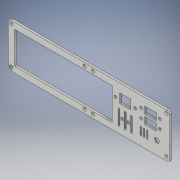
# Autodesk Inventor part: CyberDeckIOPanel2
Saved by Autodesk Inventor 2019.4 (Build 234330000, 330)
## iProperties
Created: 2020-07-26
Part Number: CyberDeckIOPanel2
Material: Generic
Document SubType Name: Modeling
Designer: Briti
Density: 1 g/cm^3
Appearance: Default
Author: Briti
Autodesk Inventor part; units mm, degrees
ref_plane "YZ Plane" through (0, 0, 0) normal (1, 0, 0) x (0, 1, 0)
ref_plane "XZ Plane" through (0, 0, 0) normal (0, 1, 0) x (-1, 0, 0)
ref_plane "XY Plane" through (0, 0, 0) normal (0, 0, 1) x (1, 0, 0)
sketch "Sketch1" plane through (0, 0, 0) normal (0, 0, 1) x (1, 0, 0)
  line L0 (-116.5, -32) -> (116.5, -32)
  line L1 (116.5, -32) -> (116.5, 32)
  line L2 (116.5, 32) -> (-116.5, 32)
  line L3 (-116.5, 32) -> (-116.5, -32)
  line L4 (-116.5, -32) -> (116.5, 32) construction
  line L5 (116.5, -32) -> (-116.5, 32) construction
  point P0 (0, 0)
  dimension "d0" = 233
  dimension "d1" = 64
  constraints: 12 end point, 2 midpoint, 2 parallel, 1 horizontal, 1 perpendicular
  measures "d0" distance of L2.end L1.end
  measures "d1" distance of L0.end L1.end
extrude "Extrusion1" add sketch "Sketch1" along normal blind 3
sketch "Sketch2" plane through (0, 0, 3) normal (0, 0, 1) x (1, 0, 0)
  arc A0 (-112, 32) -> (-116.5, 27.5) centre (-112, 27.5) ccw
  line L0 (116.5, 32) -> (-116.5, 32) projected
  line L1 (-116.5, 32) -> (-116.5, -32) projected
  arc A1 (116.5, 27.5) -> (112, 32) centre (112, 27.5) ccw
  line L2 (116.5, -32) -> (116.5, 32) projected
  line L3 (-112, 27.5) -> (-112, -26.5) construction
  line L4 (-116.5, -32) -> (116.5, -32) construction
  line L5 (-112, -26.5) -> (-107.482, -26.5) construction
  line L6 (-107.482, -26.5) -> (-107.482, -22) construction
  line L7 (-107.5, -22) -> (107.5, -22) construction
  line L8 (107.5, -22) -> (107.5, 23) construction
  line L9 (107.5, 23) -> (-107.5, 23) construction
  line L10 (-107.5, 23) -> (-107.5, -22) construction
  line L11 (-107.5, -22) -> (107.5, 23) construction
  line L12 (107.5, -22) -> (-107.5, 23) construction
  point P0 (0, 0)
  point P1 (0, 0.5)
  dimension "d4" = 9
  dimension "d5" = 9
  dimension "d6" = 54
  dimension "d7" = 4.518
  dimension "d8" = 4.5
  dimension "d9" = 215
  dimension "d10" = 45
  dimension "d11" = 9
  dimension "d12" = 9
  dimension "d13" = 9
  constraints: 18 end point, 4 point on circle, 4 point on line, 4 tangent, 2 centre point, 2 horizontal, 2 midpoint, 2 parallel, 2 perpendicular, 1 vertical
  measures "d4" diameter of A0
  measures "d5" diameter of A1
  measures "d6" distance of L3.start L3.end
  measures "d7" distance of L3.end L5.end
  measures "d8" distance of L5.end L6.end
  measures "d9" distance of L9.end L8.end
  measures "d10" distance of L8.end L7.end
  measures "d11" distance between parallel lines of L2 L8
  measures "d12" distance between parallel lines of L10 L1
  measures "d13" distance between parallel lines of L9 L0
extrude "Extrusion2" cut sketch "Sketch2" against normal blind 5
sketch "Sketch6" plane through (0, 0, 3) normal (0, 0, 1) x (1, 0, 0)
  line L0 (107.5, -22) -> (-107.5, -22) construction
  line L1 (-107.5, -22) -> (-116.5, -22) construction
  line L2 (-116.5, 27.5) -> (-116.5, -32) construction
  line L3 (-107.5, -22) -> (-107.5, -32) construction
  line L4 (-116.5, -32) -> (116.5, -32) construction
  arc A0 (-116.5, -27) -> (-111.5, -32) centre (-111.5, -27) ccw
  line L5 (-111.5, -32) -> (-116.5, -32)
  line L6 (-116.5, -32) -> (-116.5, -27)
  point P0 (0, 0)
  dimension "d32" = 10
  constraints: 8 end point, 4 point on line, 2 perpendicular, 2 point on circle, 2 tangent, 1 centre point, 1 collinear, 1 horizontal
  measures "d32" diameter of A0
extrude "Extrusion6" cut sketch "Sketch6" against normal blind 5
sketch "Sketch7" plane through (0, 0, 3) normal (0, 0, 1) x (1, 0, 0)
  arc A0 (-112, 32) -> (-116.5, 27.5) centre (-112, 27.5) ccw projected
  circle A1 centre (-112, 27.5) radius 2.4
  arc A2 (116.5, 27.5) -> (112, 32) centre (112, 27.5) ccw projected
  circle A3 centre (112, 27.5) radius 2.4
  point P0 (0, 0)
  dimension "d35" = 4.8
  dimension "d36" = 4.8
  constraints: 2 centre point, 2 coincident
  measures "d35" diameter of A1
  measures "d36" diameter of A3
extrude "Extrusion7" cut sketch "Sketch7" against normal blind 5
sketch "Sketch8" plane through (0, 0, 3) normal (0, 0, 1) x (1, 0, 0)
  arc A0 (-116.5, -27) -> (-111.5, -32) centre (-111.5, -27) ccw construction
  line L0 (-116.5, -27) -> (-116.5, -23.25) construction
  line L1 (-116.5, 27.5) -> (-116.5, -27) construction
  line L2 (-111.5, -32) -> (-107.75, -32) construction
  line L3 (-111.5, -32) -> (116.5, -32) construction
  arc A1 (-116.5, -23.25) -> (-107.75, -32) centre (-106.5699, -22.0699) ccw
  line L4 (-116.5, -23.25) -> (-116.5, -27)
  line L5 (-107.75, -32) -> (-111.5, -32)
  arc A2 (-116.5, -27) -> (-111.5, -32) centre (-111.5, -27) ccw
  point P0 (0, 0)
  dimension "d39" = 3.75
  dimension "d40" = 3.75
  dimension "d41" = 10
  constraints: 8 end point, 4 point on circle, 2 centre point, 2 collinear, 2 point on line, 1 concentric
  measures "d39" distance of L0.start L0.end
  measures "d40" distance of L2.start L2.end
  measures "d41" radius of A1
extrude "Extrusion8" cut sketch "Sketch8" against normal blind 5
sketch "Sketch9" plane through (0, 0, 3) normal (0, 0, 1) x (1, 0, 0)
  line L0 (-107.5, -22) -> (107.5, -22) construction
  line L1 (107.5, -22) -> (107.5, -32) construction
  line L2 (-107.75, -32) -> (116.5, -32) construction
  line L3 (107.5, -22) -> (120.5, -22) construction
  line L4 (107.5, -32) -> (111.5, -32) construction
  line L5 (120.5, -22) -> (120.5, -23) construction
  arc A0 (111.5, -32) -> (120.5, -23) centre (110.5456, -22.0456) ccw construction
  line L6 (116.5, -32) -> (116.5, 27.5) projected
  arc A1 (111.5, -32) -> (116.5, -30.0797) centre (110.5456, -22.0456) ccw
  line L7 (116.5, -30.0797) -> (116.5, -32)
  line L8 (111.5, -32) -> (116.5, -32)
  point P0 (0, 0)
  dimension "d44" = 13
  dimension "d45" = 4
  dimension "d46" = 1
  dimension "d47" = 10
  constraints: 12 end point, 5 point on circle, 3 point on line, 2 centre point, 2 collinear, 2 vertical, 1 concentric, 1 perpendicular
  measures "d44" distance of L0.end L3.end
  measures "d45" distance of L1.end L4.end
  measures "d46" distance of L3.end L5.end
  measures "d47" radius of A0
extrude "Extrusion9" cut sketch "Sketch9" against normal blind 5
sketch "Sketch10" plane through (0, 0, 3) normal (0, 0, 1) x (1, 0, 0)
  circle A0 centre (5.75, 27.5) radius 2.4
  line L0 (112, 32) -> (-112, 32) projected
  line L1 (-107.5, 23) -> (107.5, 23) projected
  circle A1 centre (112, 27.5) radius 2.4 projected
  circle A2 centre (-6.25, 27.5) radius 2.4
  circle A3 centre (5.75, -26.5) radius 2.4
  circle A4 centre (-6.25, -26.5) radius 2.4
  point P0 (0, 0)
  dimension "d50" = 4.8
  dimension "d51" = 4.5
  dimension "d52" = 4.5
  dimension "d53" = 106.25
  dimension "d54" = 4.8
  dimension "d55" = 12
  dimension "d56" = 4.8
  dimension "d57" = 54
  dimension "d58" = 4.8
  dimension "d59" = 12
  constraints: 4 centre point, 2 horizontal alignment, 1 vertical alignment
  measures "d50" diameter of A0
  measures "d51" distance from line of L0 A0.centre
  measures "d52" distance from line of L1 A0.centre
  measures "d53" distance of A1.centre A0.centre
  measures "d54" diameter of A2
  measures "d55" distance of A0.centre A2.centre
  measures "d56" diameter of A3
  measures "d57" distance of A3.centre A0.centre
  measures "d58" diameter of A4
  measures "d59" distance of A3.centre A4.centre
extrude "Extrusion10" cut sketch "Sketch10" against normal blind 5 contours A0 | A2 | A3 | A4
sketch "Sketch11" plane through (0, 0, 3) normal (0, 0, 1) x (1, 0, 0)
  circle A0 centre (112, -26.4995) radius 2.4
  circle A1 centre (112, 27.5) radius 2.4 construction
  circle A2 centre (112, 27.5) radius 2.4 construction
  circle A3 centre (112, -26.4995) radius 4.5 construction
  line L0 (-107.5, -22) -> (107.5, -22) construction
  line L1 (107.5, -22) -> (112.0687, -22) construction
  line L2 (107.5, -22) -> (107.5, 23) construction
  line L3 (107.5, -22) -> (107.5, -26.4995) construction
  point P0 (0, 0)
  dimension "d62" = 4.8
  dimension "d63" = 9
  constraints: 4 end point, 3 centre point, 2 coincident, 2 point on circle, 1 collinear, 1 tangent, 1 vertical alignment
  measures "d62" diameter of A0
  measures "d63" diameter of A3
extrude "Extrusion11" cut sketch "Sketch11" against normal blind 5
sketch "Sketch12" plane through (0, 0, 3) normal (0, 0, 1) x (1, 0, 0)
  line L0 (-107.5, -22) -> (107.5, -22) construction
  line L1 (-107.5, -22) -> (-116.5, -22) construction
  line L2 (-116.5, 27.5) -> (-116.5, -23.25) construction
  arc A0 (-116.5, -23.25) -> (-107.75, -32) centre (-106.5699, -22.0699) ccw construction
  line L3 (-107.5, -22) -> (-107.75, -32) construction
  circle A1 centre (-112.1139, -26.5) radius 4.5 construction
  circle A2 centre (-112.1139, -26.5) radius 2.4
  point P0 (0, 0)
  dimension "d66" = 9
  dimension "d67" = 4.8
  constraints: 4 end point, 2 centre point, 2 tangent, 1 coincident, 1 horizontal, 1 point on line
  measures "d66" diameter of A1
  measures "d67" diameter of A2
extrude "Extrusion12" cut sketch "Sketch12" against normal blind 5
sketch "Sketch22" plane through (0, 0, 0) normal (0, 0, -1) x (-1, 0, 0)
  line L0 (107.75, -32) -> (-111.5, -32) construction
  line L1 (-116.5, 32) -> (-107.5, 32) construction
  line L2 (-107.5, 32) -> (-107.5, -32) construction
  line L3 (-107.5, -32) -> (-116.5, -32) construction
  line L4 (-116.5, -32) -> (-116.5, 32) construction
  line L5 (116.5, 27.5) -> (116.5, -23.25) construction
  line L6 (-116.5, -32) -> (116.5, -32) construction
  line L7 (116.5, -32) -> (116.5, -23) construction
  line L8 (116.5, -23) -> (-116.5, -23) construction
  line L9 (-116.5, -23) -> (-116.5, -32) construction
  line L10 (-112, 32) -> (112, 32) construction
  line L11 (116.5, -32) -> (107.5, -32) construction
  line L12 (107.5, -32) -> (107.5, 32) construction
  line L13 (107.5, 32) -> (116.5, 32) construction
  line L14 (116.5, 32) -> (116.5, -32) construction
  line L15 (-116.5, -30.0797) -> (-116.5, 27.5) construction
  line L16 (116.5, 32) -> (-116.5, 32) construction
  line L17 (-116.5, 32) -> (-116.5, 23) construction
  line L18 (-116.5, 23) -> (116.5, 23) construction
  line L19 (116.5, 23) -> (116.5, 32) construction
  line L20 (-107.5, 23) -> (-107.5, 16) construction
  line L21 (-107.5, 16) -> (-102.5, 16) construction
  circle A0 centre (-102.5, 16) radius 5 construction
  line L22 (-97.5, 16) -> (-80.5, 16) construction
  line L23 (-80.5, 16) -> (-75.5, 16) construction
  circle A1 centre (-75.5, 16) radius 5 construction
  line L24 (-80.5, 10) -> (-97.5, 10) construction
  line L25 (-97.5, 10) -> (-97.5, 22) construction
  line L26 (-97.5, 22) -> (-80.5, 22) construction
  line L27 (-80.5, 22) -> (-80.5, 10) construction
  line L28 (-80.5, 10) -> (-97.5, 22) construction
  line L29 (-97.5, 10) -> (-80.5, 22) construction
  line L30 (-97.5, 22) -> (-99.5, 22) construction
  line L31 (-99.5, 22) -> (-99.5, 10) construction
  line L32 (-99.5, 10) -> (-97.5, 9) construction
  line L33 (-80.5, 22) -> (-78.5, 22) construction
  line L34 (-78.5, 22) -> (-78.5, 10) construction
  line L35 (-78.5, 10) -> (-80.5, 10) construction
  line L36 (-97.5, 11) -> (-80.5, 11)
  line L37 (-80.5, 11) -> (-80.5, 21)
  line L38 (-80.5, 21) -> (-97.5, 21)
  line L39 (-97.5, 21) -> (-97.5, 11)
  line L40 (-97.5, 11) -> (-80.5, 21) construction
  line L41 (-80.5, 11) -> (-97.5, 21) construction
  circle A2 centre (-102.5, 16) radius 2
  circle A3 centre (-75.5, 16) radius 2
  line L42 (-97.5, 9) -> (-80.5, 9) construction
  line L43 (-80.5, 9) -> (-80.5, -3) construction
  line L44 (-80.5, -3) -> (-97.5, -3) construction
  line L45 (-97.5, -3) -> (-97.5, 9) construction
  line L46 (-97.5, 3) -> (-102.5, 3) construction
  line L47 (-80.5, 3) -> (-75.5, 3) construction
  circle A4 centre (-102.5, 3) radius 5 construction
  circle A5 centre (-75.5, 3) radius 5 construction
  line L48 (-97.5, 9) -> (-99.5, 10) construction
  line L49 (-99.5, 10) -> (-99.5, -3) construction
  line L50 (-99.5, -3) -> (-97.5, -3) construction
  line L51 (-80.5, -3) -> (-78.5, -3) construction
  line L52 (-78.5, -3) -> (-78.5, 10) construction
  line L53 (-78.5, 10) -> (-80.5, 10) construction
  line L54 (-89, 9) -> (-89, -3) construction
  line L55 (-97.5, 3) -> (-80.5, 3) construction
  line L56 (-97.5, -2) -> (-80.5, -2)
  line L57 (-80.5, -2) -> (-80.5, 8)
  line L58 (-80.5, 8) -> (-97.5, 8)
  line L59 (-97.5, 8) -> (-97.5, -2)
  line L60 (-97.5, -2) -> (-80.5, 8) construction
  line L61 (-80.5, -2) -> (-97.5, 8) construction
  circle A6 centre (-102.5, 3) radius 2
  circle A7 centre (-75.5, 3) radius 2
  line L62 (-89, -3) -> (-89, -23) construction
  line L63 (-89, -13) -> (-107.5, -13) construction
  line L64 (-70.5, 16) -> (-70.5, 23) construction
  line L65 (-70.5, 16) -> (-70.5, -23) construction
  line L66 (-89, -13) -> (-70.5, -13) construction
  circle A8 centre (-98.25, -13) radius 3.5
  line L67 (-79.75, -18) -> (-79.75, -8) construction
  line L68 (-78.75, -18) -> (-78.75, -8)
  line L69 (-80.75, -8) -> (-80.75, -18)
  arc A9 (-80.75, -18) -> (-78.75, -18) centre (-79.75, -18) ccw
  arc A10 (-78.75, -8) -> (-80.75, -8) centre (-79.75, -8) ccw
  line L70 (-89, -13) -> (-79.75, -13) construction
  line L71 (-79.75, -13) -> (-70.5, -13) construction
  line L72 (-84.375, -18) -> (-84.375, -8) construction
  line L73 (-83.375, -18) -> (-83.375, -8)
  line L74 (-85.375, -8) -> (-85.375, -18)
  arc A11 (-85.375, -18) -> (-83.375, -18) centre (-84.375, -18) ccw
  arc A12 (-83.375, -8) -> (-85.375, -8) centre (-84.375, -8) ccw
  line L75 (-75.125, -18) -> (-75.125, -8) construction
  line L76 (-74.125, -18) -> (-74.125, -8)
  line L77 (-76.125, -8) -> (-76.125, -18)
  arc A13 (-76.125, -18) -> (-74.125, -18) centre (-75.125, -18) ccw
  arc A14 (-74.125, -8) -> (-76.125, -8) centre (-75.125, -8) ccw
  point P0 (0, 0)
  point P1 (-89, 16)
  point P2 (-89, 3)
  point P3 (-84.375, -13)
  point P4 (-75.125, -13)
  dimension "d172" = 9
  dimension "d173" = 9
  dimension "d174" = 9
  dimension "d175" = 9
  dimension "d176" = 7
  dimension "d177" = 5
  dimension "d178" = 17
  dimension "d179" = 5
  dimension "d180" = 12
  dimension "d181" = 2
  dimension "d182" = 2
  dimension "d183" = 17
  dimension "d184" = 10
  dimension "d185" = 4
  dimension "d186" = 4
  dimension "d187" = 12
  dimension "d188" = 5
  dimension "d189" = 5
  dimension "d190" = 2
  dimension "d191" = 17
  dimension "d192" = 10
  dimension "d193" = 4
  dimension "d194" = 4
  dimension "d195" = 7
  dimension "d196" = 5
  dimension "d197" = 2
  dimension "d198" = 5
  dimension "d199" = 2
  dimension "d200" = 5
  dimension "d201" = 2
  dimension "d204" = 37
  constraints: 154 end point, 21 parallel, 20 midpoint, 20 perpendicular, 18 point on line, 16 point on circle, 13 centre point, 13 horizontal, 13 tangent, 8 coincident, 3 collinear, 2 horizontal alignment, 4 other
  measures "d172" distance of L2.end L3.end
  measures "d173" distance of L7.end L6.end
  measures "d174" distance of L12.end L13.end
  measures "d175" distance of L17.end L16.end
  measures "d176" distance of L20.start L20.end
  measures "d177" distance of L20.end L21.end
  measures "d178" distance of L22.start L22.end
  measures "d179" distance of L22.end L23.end
  measures "d180" distance of L24.end L25.end
  measures "d181" distance of L25.end L30.end
  measures "d182" distance of L26.end L33.end
  measures "d183" distance of L38.end L37.end
  measures "d184" distance of L37.end L36.end
  measures "d185" diameter of A2
  measures "d186" diameter of A3
  measures "d187" distance of L42.end L43.end
  measures "d188" distance of L46.start L46.end
  measures "d189" distance of L47.start L47.end
  measures "d190" distance of L43.end L51.end
  measures "d191" distance of L58.end L57.end
  measures "d192" distance of L57.end L56.end
  measures "d193" diameter of A6
  measures "d194" diameter of A7
  measures "d195" diameter of A8
  measures "d196" distance of L70.end L67.end
  measures "d197" diameter of A10
  measures "d198" distance of point (-84.375, -13) L72.end
  measures "d199" diameter of A12
  measures "d200" distance of point (-75.125, -13) L75.end
  measures "d201" diameter of A14
  measures "d204" distance of L20.start L64.end
extrude "Extrusion18" cut sketch "Sketch22" against normal blind 20
sketch "Sketch23" plane through (0, 0, 0) normal (0, 0, -1) x (-1, 0, 0)
  line L0 (-112, 32) -> (112, 32) construction
  line L1 (-116.5, -32) -> (-107.5, -32) construction
  line L2 (-107.5, -32) -> (-107.5, 32) construction
  line L3 (-107.5, 32) -> (-116.5, 32) construction
  line L4 (-116.5, 32) -> (-116.5, -32) construction
  line L5 (116.5, 27.5) -> (116.5, -23.25) construction
  line L6 (-116.5, 32) -> (116.5, 32) construction
  line L7 (116.5, 32) -> (116.5, 23) construction
  line L8 (116.5, 23) -> (-116.5, 23) construction
  line L9 (-116.5, 23) -> (-116.5, 32) construction
  line L10 (107.75, -32) -> (-111.5, -32) construction
  line L11 (116.5, 23) -> (107.5, 23) construction
  line L12 (107.5, 23) -> (107.5, -32) construction
  line L13 (107.5, -32) -> (116.5, -32) construction
  line L14 (116.5, -32) -> (116.5, 23) construction
  line L15 (-116.5, -30.0797) -> (-116.5, 27.5) construction
  line L16 (116.5, -32) -> (-116.5, -32) construction
  line L17 (-116.5, -32) -> (-116.5, -23) construction
  line L18 (-116.5, -23) -> (116.5, -23) construction
  line L19 (116.5, -23) -> (116.5, -32) construction
  line L20 (-107.5, 23) -> (-70.5, 23) construction
  line L21 (-70.5, 23) -> (-70.5, -23) construction
  circle A0 centre (-98.25, -13) radius 3.5 projected
  circle A1 centre (-98.25, -13) radius 5
  point P0 (0, 0)
  dimension "d205" = 9
  dimension "d206" = 9
  dimension "d207" = 9
  dimension "d208" = 9
  dimension "d209" = 37
  dimension "d210" = 10
  constraints: 36 end point, 8 parallel, 8 point on line, 5 perpendicular, 4 horizontal, 1 centre point, 1 coincident
  measures "d205" distance of L3.end L2.end
  measures "d206" distance of L6.end L7.end
  measures "d207" distance of L13.end L12.end
  measures "d208" distance of L16.end L17.end
  measures "d209" distance of L20.start L20.end
  measures "d210" diameter of A1
extrude "Extrusion19" cut sketch "Sketch23" against normal blind 1.5
sketch "Sketch24" plane through (0, 0, 0) normal (0, 0, -1) x (-1, 0, 0)
  line L0 (116.5, 27.5) -> (116.5, -23.25) construction
  line L1 (-116.5, 32) -> (116.5, 32) construction
  line L2 (116.5, 32) -> (116.5, 23) construction
  line L3 (116.5, 23) -> (-116.5, 23) construction
  line L4 (-116.5, 23) -> (-116.5, 32) construction
  line L5 (107.75, -32) -> (-111.5, -32) construction
  line L6 (116.5, 32) -> (107.5, 32) construction
  line L7 (107.5, 32) -> (107.5, -32) construction
  line L8 (107.5, -32) -> (116.5, -32) construction
  line L9 (116.5, -32) -> (116.5, 32) construction
  line L10 (-116.5, -30.0797) -> (-116.5, 27.5) construction
  line L11 (116.5, -32) -> (-116.5, -32) construction
  line L12 (-116.5, -32) -> (-116.5, -23) construction
  line L13 (-116.5, -23) -> (116.5, -23) construction
  line L14 (116.5, -23) -> (116.5, -32) construction
  line L15 (-112, 32) -> (112, 32) construction
  line L16 (-116.5, -32) -> (-107.5, -32) construction
  line L17 (-107.5, -32) -> (-107.5, 32) construction
  line L18 (-107.5, 32) -> (-116.5, 32) construction
  line L19 (-116.5, 32) -> (-116.5, -32) construction
  line L20 (-107.5, 23) -> (-70.5, 23) construction
  line L21 (-70.5, 23) -> (-70.5, -23) construction
  line L22 (-70.5, 23) -> (-34.5, 23) construction
  line L23 (-34.5, 23) -> (-34.5, -23) construction
  line L24 (-34.5, 23) -> (-34.5, 0) construction
  line L25 (-34.5, 0) -> (-70.5, 0) construction
  line L26 (-63, 1) -> (-42, 1) construction
  line L27 (-42, 1) -> (-42, 22) construction
  line L28 (-42, 22) -> (-63, 22) construction
  line L29 (-63, 22) -> (-63, 1) construction
  line L30 (-63, 1) -> (-42, 22) construction
  line L31 (-42, 1) -> (-63, 22) construction
  line L32 (-63, 22) -> (-63, 15) construction
  line L33 (-42, 22) -> (-42, 15) construction
  line L34 (-63, 15) -> (-70.5, 15) construction
  line L35 (-70.5, 15) -> (-70.5, 7.5) construction
  line L36 (-70.5, 7.5) -> (-63, 7.5) construction
  line L37 (-42, 15) -> (-34.5, 15) construction
  line L38 (-34.5, 15) -> (-34.5, 7.5) construction
  line L39 (-34.5, 7.5) -> (-42, 7.5) construction
  circle A0 centre (-66.75, 11.25) radius 3.75 construction
  circle A1 centre (-38.25, 11.25) radius 3.75 construction
  line L40 (-52.5, 11.5) -> (-52.5, 12.875) construction
  line L41 (-60.5, 6.25) -> (-44.5, 6.25)
  line L42 (-44.5, 6.25) -> (-44.5, 19.5)
  line L43 (-44.5, 19.5) -> (-60.5, 19.5)
  line L44 (-60.5, 19.5) -> (-60.5, 6.25)
  line L45 (-60.5, 6.25) -> (-44.5, 19.5) construction
  line L46 (-44.5, 6.25) -> (-60.5, 19.5) construction
  circle A2 centre (-66.75, 11.25) radius 2
  circle A3 centre (-38.25, 11.25) radius 2
  line L47 (-52.5, 0) -> (-52.5, -23) construction
  line L48 (-52.5, -23) -> (-70.5, -23) construction
  line L49 (-52.5, -23) -> (-34.5, -23) construction
  line L50 (-61.5, -21.5) -> (-61.5, -1.5) construction
  line L51 (-60.25, -21.5) -> (-60.25, -1.5)
  line L52 (-62.75, -1.5) -> (-62.75, -21.5)
  arc A4 (-62.75, -21.5) -> (-60.25, -21.5) centre (-61.5, -21.5) ccw
  arc A5 (-60.25, -1.5) -> (-62.75, -1.5) centre (-61.5, -1.5) ccw
  line L53 (-61.5, -11.5) -> (-41.5, -11.5) construction
  line L54 (-52.5, -21.5) -> (-52.5, -1.5) construction
  line L55 (-51, -21.5) -> (-51, -1.5)
  line L56 (-54, -1.5) -> (-54, -21.5)
  arc A6 (-54, -21.5) -> (-51, -21.5) centre (-52.5, -21.5) ccw
  arc A7 (-51, -1.5) -> (-54, -1.5) centre (-52.5, -1.5) ccw
  line L57 (-43.5, -21.5) -> (-43.5, -1.5) construction
  line L58 (-42.25, -21.5) -> (-42.25, -1.5)
  line L59 (-44.75, -1.5) -> (-44.75, -21.5)
  arc A8 (-44.75, -21.5) -> (-42.25, -21.5) centre (-43.5, -21.5) ccw
  arc A9 (-42.25, -1.5) -> (-44.75, -1.5) centre (-43.5, -1.5) ccw
  line L60 (-43.5, -11.5) -> (-23.5, -11.5) construction
  line L61 (-61.5, -11.5) -> (-52.5, -11.5) construction
  line L62 (-52.5, -11.5) -> (-43.5, -11.5) construction
  circle A10 centre (-57, -11.5) radius 2
  circle A11 centre (-48, -11.5) radius 2
  point P0 (0, 0)
  dimension "d213" = 9
  dimension "d214" = 9
  dimension "d215" = 9
  dimension "d216" = 9
  dimension "d217" = 37
  dimension "d218" = 36
  dimension "d219" = 21
  dimension "d220" = 21
  dimension "d221" = 7
  dimension "d222" = 7
  dimension "d223" = 7.5
  dimension "d224" = 1.375
  dimension "d225" = 16
  dimension "d226" = 13.25
  dimension "d227" = 4
  dimension "d228" = 4
  dimension "d231" = 10
  dimension "d232" = 90
  dimension "d233" = 2.5
  dimension "d234" = 10
  dimension "d235" = 3
  dimension "d236" = 10
  dimension "d237" = 90
  dimension "d238" = 2.5
  dimension "d239" = 4
  dimension "d240" = 4
  constraints: 124 end point, 23 point on line, 17 parallel, 13 midpoint, 13 perpendicular, 12 centre point, 12 point on circle, 12 tangent, 8 horizontal, 4 collinear, 2 coincident, 1 vertical
  measures "d213" distance of L1.end L2.end
  measures "d214" distance of L8.end L7.end
  measures "d215" distance of L11.end L12.end
  measures "d216" distance of L18.end L17.end
  measures "d217" distance of L20.start L20.end
  measures "d218" distance of L20.end L22.end
  measures "d219" distance of L28.end L27.end
  measures "d220" distance of L27.end L26.end
  measures "d221" distance of L28.end L32.end
  measures "d222" distance of L27.end L33.end
  measures "d223" distance of L34.end L35.end
  measures "d224" distance of L40.start L40.end
  measures "d225" distance of L43.end L42.end
  measures "d226" distance of L42.end L41.end
  measures "d227" diameter of A2
  measures "d228" diameter of A3
  measures "d231" distance of L53.start L50.end
  measures "d232" angle of L53 L50
  measures "d233" diameter of A5
  measures "d234" distance of L61.end L54.end
  measures "d235" diameter of A7
  measures "d236" distance of L60.start L57.end
  measures "d237" angle of L60 L57
  measures "d238" diameter of A9
  measures "d239" diameter of A10
  measures "d240" diameter of A11
extrude "Extrusion20" cut sketch "Sketch24" against normal blind 3
sketch "Sketch25" plane through (0, 0, 0) normal (0, 0, -1) x (-1, 0, 0)
  line L0 (116.5, 27.5) -> (116.5, -23.25) construction
  line L1 (-116.5, 32) -> (116.5, 32) construction
  line L2 (116.5, 32) -> (116.5, 23) construction
  line L3 (116.5, 23) -> (-116.5, 23) construction
  line L4 (-116.5, 23) -> (-116.5, 32) construction
  line L5 (107.75, -32) -> (-111.5, -32) construction
  line L6 (116.5, 32) -> (107.5, 32) construction
  line L7 (107.5, 32) -> (107.5, -32) construction
  line L8 (107.5, -32) -> (116.5, -32) construction
  line L9 (116.5, -32) -> (116.5, 32) construction
  line L10 (-116.5, -30.0797) -> (-116.5, 27.5) construction
  line L11 (116.5, -32) -> (-116.5, -32) construction
  line L12 (-116.5, -32) -> (-116.5, -23) construction
  line L13 (-116.5, -23) -> (116.5, -23) construction
  line L14 (116.5, -23) -> (116.5, -32) construction
  line L15 (-112, 32) -> (112, 32) construction
  line L16 (-116.5, -32) -> (-107.5, -32) construction
  line L17 (-107.5, -32) -> (-107.5, 32) construction
  line L18 (-107.5, 32) -> (-116.5, 32) construction
  line L19 (-116.5, 32) -> (-116.5, -32) construction
  line L20 (-107.5, 23) -> (-70.5, 23) construction
  line L21 (-70.5, 23) -> (-33.5, 23) construction
  line L22 (-33.5, 23) -> (-33.5, -23) construction
  line L23 (-33.5, 23) -> (107.5, 23)
  line L24 (107.5, 23) -> (107.5, -23)
  line L25 (107.5, -23) -> (-33.5, -23)
  line L26 (-33.5, -23) -> (-33.5, 23)
  point P0 (0, 0)
  dimension "d241" = 9
  dimension "d242" = 9
  dimension "d243" = 9
  dimension "d244" = 9
  dimension "d245" = 37
  dimension "d246" = 37
  constraints: 46 end point, 11 point on line, 10 parallel, 6 perpendicular, 5 horizontal
  measures "d241" distance of L1.end L2.end
  measures "d242" distance of L8.end L7.end
  measures "d243" distance of L11.end L12.end
  measures "d244" distance of L18.end L17.end
  measures "d245" distance of L20.start L20.end
  measures "d246" distance of L20.end L21.end
extrude "Extrusion21" cut sketch "Sketch25" against normal blind 3
body "Solid1"
